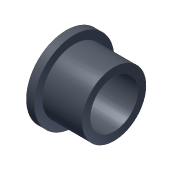
# Autodesk Inventor part: PP-00065
Saved by Autodesk Inventor 2012 (Build 160160000, 160)
## iProperties
Created: 2011-06-15
Part Number: PP-00065
Document SubType Name: Modeling
Designer: dfoster
Density: 1 g/cm^3
Description: Bushing, Flanged
Mass: 0.641005 g
Surface Area: 9.34242 cm^2
Volume: 0.641005 cm^3
Material: Default
Title: Bushing, Flanged
Author: dfoster
Autodesk Inventor part; units mm, degrees
ref_plane "YZ Plane" through (0, 0, 0) normal (1, 0, 0) x (0, 1, 0)
ref_plane "XZ Plane" through (0, 0, 0) normal (0, 1, 0) x (-1, 0, 0)
ref_plane "XY Plane" through (0, 0, 0) normal (0, 0, 1) x (1, 0, 0)
sketch "Sketch1" plane through (0, 0, 0) normal (0, 0, 1) x (1, 0, 0)
  line L0 (0, 7.9375) -> (0, 4.7625)
  line L1 (0, 4.7625) -> (9.525, 4.7625)
  line L2 (9.525, 4.7625) -> (9.525, 6.35)
  line L3 (9.525, 6.35) -> (1.5875, 6.35)
  line L4 (1.5875, 6.35) -> (1.5875, 7.9375)
  line L5 (1.5875, 7.9375) -> (0, 7.9375)
  line L6 (0, 0) -> (25.6678, 0)
  dimension "d0" = 4.7625
  dimension "d1" = 6.35
  dimension "d2" = 7.9375
  dimension "d3" = 1.5875
  dimension "d4" = 9.525
  constraints: 14 end point, 4 parallel, 1 horizontal, 1 perpendicular, 1 vertical
  measures "d0" distance from line of L6.start L1
  measures "d1" distance from line of L6.start L3
  measures "d2" distance from line of L5 L6.start
  measures "d3" distance between parallel lines of L4 L0
  measures "d4" distance of L0.end L1.end
revolve "Revolution1" add sketch "Sketch1" angle 360 about axis through (0, 0, 0) along (1, 0, 0)
body "Solid1"
